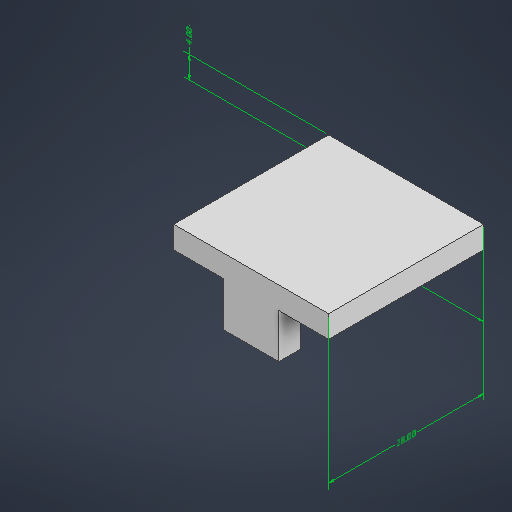
# Autodesk Inventor part: Schemo lcd
Saved by Autodesk Inventor 2026.2 (Build 302298000, 298)
## iProperties
Created: 2026-01-19
Part Number: Schemo lcd
Material: Generic
Document SubType Name: Modeling
Designer: ASUS
Density: 1 g/cm^3
Appearance: Default
Mass: 3.456 g
Surface Area: 22.4 cm^2
Volume: 3.456 cm^3
Author: ASUS
Autodesk Inventor part; units mm, degrees
ref_plane "YZ Plane" through (0, 0, 0) normal (1, 0, 0) x (0, 1, 0)
ref_plane "XZ Plane" through (0, 0, 0) normal (0, 1, 0) x (-1, 0, 0)
ref_plane "XY Plane" through (0, 0, 0) normal (0, 0, 1) x (1, 0, 0)
sketch "Sketch1" plane through (0, 0, 0) normal (0, 1, 0) x (-1, 0, 0)
  line L0 (0, 0) -> (-28, 0)
  line L1 (-28, 0) -> (-28, 28)
  line L2 (-28, 28) -> (0, 28)
  line L3 (0, 28) -> (0, 0)
  dimension "d0" = 28
  dimension "d1" = 28
  constraints: 8 end point, 2 parallel, 1 horizontal, 1 perpendicular
  measures "d0" distance of L1.end L2.end
  measures "d1" distance of L0.end L1.end
extrude "Extrusion1" add sketch "Sketch1" along normal blind 4
sketch "Sketch2" plane through (0, 0, 0) normal (0, -1, 0) x (1, 0, 0)
  line L0 (0, 28) -> (28, 28) projected
  line L1 (14, 28) -> (19, 28)
  line L2 (19, 28) -> (19, 24)
  line L3 (19, 24) -> (9, 24)
  line L4 (9, 24) -> (9, 28)
  point P0 (0, 0)
  dimension "d6" = 5
  dimension "d7" = 4
  dimension "d8" = 10
  constraints: 8 end point, 3 perpendicular, 2 point on line
  measures "d6" distance of L1.start L1.end
  measures "d7" distance of L1.end L2.end
  measures "d8" distance of L2.end L3.end
extrude "Extrusion2" add sketch "Sketch2" along normal blind 8
body "Solid1"
